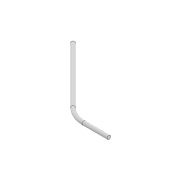
# Autodesk Inventor part: cable
Saved by Autodesk Inventor 2022 (Build 260153000, 153)
## iProperties
Created: 2022-11-22
Part Number: cable
Material: Generic
Document SubType Name: Modeling
Designer: kylem
Density: 1 g/cm^3
Appearance: Default
Author: kylem
Autodesk Inventor part; units mm, degrees
ref_plane "YZ Plane" through (0, 0, 0) normal (1, 0, 0) x (0, 1, 0)
ref_plane "XZ Plane" through (0, 0, 0) normal (0, 1, 0) x (-1, 0, 0)
ref_plane "XY Plane" through (0, 0, 0) normal (0, 0, 1) x (1, 0, 0)
sketch "Sketch1" plane through (0, 0, 0) normal (0, 1, 0) x (-1, 0, 0)
  line L0 (0, 0) -> (33.5434, 0)
  line L1 (60, 0) -> (29.825, 0) construction
  arc A0 (20.1723, -0.0304) -> (19.825, 0) centre (19.825, -2) ccw
  line L2 (58.2922, -10.2513) -> (133.4916, -85.4506)
  line L3 (62.7809, -14.74) -> (169.1289, -14.74) construction
  arc A1 (58.2922, -10.2513) -> (33.5434, 0) centre (33.5434, -35) ccw
  point P0 (16.6863, 0)
  dimension "d0" = 60
  dimension "d1" = 15
  dimension "d5" = 2
  dimension "d12" = 100
  dimension "d13" = 45
  dimension "d14" = 35
  constraints: 8 end point, 4 point on circle, 4 point on line, 3 horizontal, 3 tangent, 2 centre point, 1 equal length
  measures "d0" distance of L0.start L1.start
  measures "d1" distance of L1.start L3.start
  measures "d5" radius of A0
  measures "d12" distance of L3.start L2.end
  measures "d13" angle of L2 L3
  measures "d14" radius of A1
sketch "Sketch2" plane through (0, 0, 0) normal (1, 0, 0) x (0, 1, 0)
  circle A0 centre (0, 0) radius 2.5
  dimension "d9" = 5
  constraints: 1 centre point, 1 coincident
  measures "d9" diameter of A0
sweep "Sweep1" add profiles "Sketch2" path "Sketch1" path curves L0 A1 L2
body "Solid1"
